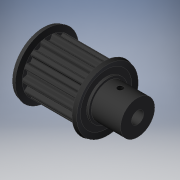
# Autodesk Inventor part: TTPA14T5200-B-P5_b
Saved by Autodesk Inventor 2019 (Build 230136000, 136)
## iProperties
Created: 2023-11-07
Part Number: TTPA14T5200-B-P5_b
Material: Generic
Catalog Web Link: www.cadenas.de
Description: TTPA__T5050, TTPA__T5100, TTPA__T5150, TTPA__T5200, TTPA__T5250, TTPB__T5050, TTPB__T5100, TTPB__T5150, TTPB__T5200, TTPB__T5250, TTPK__T5050, TTPK__T5100, TTPK__T5150, TTPK__T5200, TTPK__T5250, TTPN__T5050, TTPN__T5100, TTPN__T5150, TTPN__T5200, TTPN__T5250, TTPT__T5050, TTPT__T5100, TTPT__T5150, TTPT__T5200, TTPT__T5250, TTPM__T5050, TTPM__T5100, TTPM__T5150, TTPM__T5200, TTPM__T5250, TTPP__T5050, TTPP__T5100, TTPP__T5150, TTPP__T5200, TTPP__T5250, TTPS__T5050, TTPS__T5100, TTPS__T5150, TTPS__T5200, TTPS__T5250_b-Timing Pulleys T5 Type
Vendor: MISUMI
Document SubType Name: Modeling
Designer: psAdmin
Manufacturer: MISUMI
Mass: 9.71654 g
Surface Area: 50.0601 cm^2
Volume: 9.71654 cm^3
Density: 1 g/cm^3
Appearance: PSOLRGB-175-175-175
Category: PARTsolutions
Company: MISUMI
Title: TTPA14T5200-B-P5
Author: Cadenas PARTsolutions
Comments: Timing Pulleys T5 Type
PSOL_IDENT_0: {$CADENAS_DATA/23d-libs/misumi/metric/51_timing_pulleys/ttpt_t5/ttpa_t5.prj},938 {VTYP=3D},{NB=TTPA1
PSOL_IDENT_1: 4T5200-B-P5_b},{LINA=TTPA14T5200-B-P5},{NN=TTPA__T5050, TTPA__T5100, TTPA__T5150, TTPA__T5200, TTPA_
PSOL_IDENT_2: _T5250, TTPB__T5050, TTPB__T5100, TTPB__T5150, TTPB__T5200, TTPB__T5250, TTPK__T5050, TTPK__T5100, T
PSOL_IDENT_3: TPK__T5150, TTPK__T5200, TTPK__T5250, TTPN__T5050, TTPN__T5100, TTPN__T5150, TTPN__T5200, TTPN__T525
PSOL_IDENT_4: 0, TTPT__T5050, TTPT__T5100, TTPT__T5150, TTPT__T5200, TTPT__T5250, TTPM__T5050, TTPM__T5100, TTPM__
PSOL_IDENT_5: T5150, TTPM__T5200, TTPM__T5250, TTPP__T5050, TTPP__T5100, TTPP__T5150, TTPP__T5200, TTPP__T5250, TT
PSOL_IDENT_6: PS__T5050, TTPS__T5100, TTPS__T5150, TTPS__T5200, TTPS__T5250_b},{DATE=29.05.2023 09:16:51},{GEOMDAT
PSOL_IDENT_7: E=15.12.2022 08:47:30},{VERSION=},{LINEID=320},{WBVAR=MATP,ST,TNW,PS,SBS,DD,Z,J,Q,R,S,T,ALT1,ALT2,M,
PSOL_IDENT_8: QSC,QFC,QTC,ALT3,K,KSC,KFC,KTC,ALT4,ZM,ZSC,ZFC,ZTC,ALT5,ALT6,ALT7,FC,ALT8,SRG,ALT9,BTC,TL,ALT10,TPC,
PSOL_IDENT_9: ALT11,BC,ALT12,SLH,ALT13,BN},{WBNUMERIC=DD,Z,J,Q,R,S,T,QSC,QFC,QTC,K,KSC,KFC,KTC,ZSC,ZFC,ZTC,FC,SRG,
PSOL_IDENT_10: BTC,TL,BC,SLH,BN}  {NB=TTPA14T5200-B-P5_b},{LINA=TTPA14T5200-B-P5},{KT=DUMMY},{PN=TTPA14T5200-B-P5},
PSOL_IDENT_11: {TYPE=TTPA},{MATP=A2017},{MATPALG= 'A2017','Aluminum Alloy 2000 series','S45C','1045 Carbon Steel Eq
PSOL_IDENT_12: uivalent','SUS304','304 Stainless Steel' },{ST=CA},{STALG= 'CA','Clear Anodize','BA','Black Anodize'
PSOL_IDENT_13: ,'HAT','Hard Clear Anodize','ENP','Electroless Nickel Plating' },{NT=14},{TNW=T5200},{TNWALG= 'T5050'
PSOL_IDENT_14: , 'T5100' , 'T5150' , 'T5200' , 'T5250' },{BW=20},{PS=B},{PSALG= 'A','B' },{SBS=P},{SBSALG= 'H','Ro
PSOL_IDENT_15: und Hole','P','Round Hole + Tap','V','Stepped Hole','F','Stepped Hole (Counterbore holes on the boss
PSOL_IDENT_16: side)' },{DD=5.00},{DDALG=[5:6/1],6.35,[7:8/1]},{DDHA=},{DDPA=},{DDNA=},{DDCA=},{DDVA=},{DDY=},{DDW
PSOL_IDENT_17: B=},{DDHB=[5:6/1],6.35,[7:10/1]},{DDPB=[5:6/1],6.35,[7:8/1]},{DDNB=},{DDNK=[10:10/1]},{DDCB=},{DDVFB=
PSOL_IDENT_18: [5:6/1],6.35,[7:8/1]},{Z=0},{ZALG=[0]},{ZMIN=7.000},{ZAMAX=0.000},{ZBMAX=10.000},{DDZ=5.000},{J=0.0}
PSOL_IDENT_19: ,{JALG=[0]},{JMIN=2.000},{JMAX=37.000},{JPN=},{Q=0},{QALG=[0]},{QRMIN=7.000},{QRMAX=0.000},{WBQMIN=9
PSOL_IDENT_20: .000},{R=0},{RALG=[0]},{WBRMAX=-2.000},{S=0.0},{SALG=[0]},{SMAX=14.000},{T=0.0},{TALG=[0]},{TMAX=14.
PSOL_IDENT_21: 000},{SBSPN=-P5},{A=22},{W=27},{L=39},{PD=22.28},{OD=21.45},{D=14},{DALG=14.000},{DE=14.000},{F=26},
PSOL_IDENT_22: {E=16},{TT=1.6},{BBK=0.000},{TTK=0.000},{ALT1=},{ALT1ALG= '','w/o KC90 (Set Screw Angle)','KC90','wi
PSOL_IDENT_23: th KC90 (Set Screw Angle)' },{ANG=120.000},{ALT1PN=},{ALT2=},{ALT2ALG= '','Not applicable' },{M=N/A}
PSOL_IDENT_24: ,{MALG= 'N/A' },{MFTALG= 'N/A' },{MSALG= 'N/A' },{M3D=0.000},{KDML=0.000},{ML=0.000},{MUL=0.000},{PI
PSOL_IDENT_25: TCH=0.000},{QSC=0.0},{QSCALG=0},{QFC=0.0},{QFCALG=0},{QTC=0.0},{QTCALG=0},{QPCDMIN=0.000},{QPCDMINAL
PSOL_IDENT_26: G=0.000},{QPCDMAX=10.000},{ALT2PN=},{TAP=0.000},{ALT3=},{ALT3ALG= '','Not applicable' },{K=0.0},{KAL
PSOL_IDENT_27: G=0},{KMIN=4.000},{KFTMAX=0.000},{KSMAX=0.000},{KSC=0.0},{KSCALG=0},{KFC=0.0},{KFCALG=0},{KTC=0.0},{
PSOL_IDENT_28: KTCALG=0},{KSCMIN=9.000},{KPCDMIN=9.000},{KPCDMAX=10.000},{ALT3PN=},{ALT4=},{ALT4ALG= '','Not applic
PSOL_IDENT_29: able' },{ALT4MIN=15.500},{ALT4MAX=5.500},{ZM=N/A},{ZMALG= 'N/A' },{ZMFTALG= 'N/A' },{ZMSALG= 'N/A' }
PSOL_IDENT_30: ,{ZMDD1=0.0},{ZMDD2=0.0},{ZMHH=0.0},{ZSC=0.0},{ZSCALG=[0]},{ZFC=0.0},{ZFCALG=[0]},{ZTC=0.0},{ZTCALG=
PSOL_IDENT_31: [0]},{ZPCDMIN=0.000},{ZPCDMINALG=0.000},{ZPCDMAX=10.000},{ALT4PN=},{ALT5=},{ALT5ALG= '','w/o Flange
PSOL_IDENT_32: not Attached','NFC','with NFC (Flange not Attached)' },{ALT5PN=},{ALT6=},{ALT6ALG= '','w/o Flange At
PSOL_IDENT_33: tached on One Side Only','RFC','with RFC (Flange Attached on The Boss Side Only)','LFC','with LFC (F
PSOL_IDENT_34: lange Attached on The Opposite Side Only)' },{ALT6PN=},{ALT7=},{ALT7ALG= '','w/o FC (Flange Cut)','F
PSOL_IDENT_35: C','with FC (Flange Cut)' },{FC=0.0},{FCALG=0},{FCMIN=22.5},{FCMAX=24.0},{ALT7PN=},{ALT8=},{ALT8ALG=
PSOL_IDENT_36: '','Not applicable' },{ALT8ALGALG=10.000},{ALT8DD2=0.000},{ALT8MM=0.000},{ALT8NN=0.000},{QC=0.000},
PSOL_IDENT_37: {KC=0.000},{ZC=0.000},{SRG=0.0},{SRGALG=[0]},{SRGMAX=0.000},{SRGMAX1=0.000},{DD2=0.0},{MM=0.00},{NN=
PSOL_IDENT_38: 0.00},{ALT8PN=},{ALT9=},{ALT9ALG= '','Not applicable' },{BTC9=7.000},{TL9=1.000},{BTC=0},{BTCALG=[0]
PSOL_IDENT_39: },{TL=0.0},{TLALG=0},{TLMIN=1.000},{TLMAX=-27.500},{BTCL=0},{BTCD=0},{ALT9PN=},{WLBCTL=39.000},{ALT1
PSOL_IDENT_40: 0=},{ALT10ALG= '','w/o TPC (Tapped Hole Dimension)','TPC','with TPC (Tapped Hole Dimension)' },{TPC=
PSOL_IDENT_41: N/A},{TPCALG= 'N/A' },{TPCM=3.000},{ALT10PN=},{ALT11=},{ALT11ALG= '','w/o BC (Boss Cut)','BC','with
PSOL_IDENT_42: BC (Boss Cut)' },{BC=0.0},{BCALG=0},{BCMIN=6.000},{BCMAX=11.500},{M1WBC=32.000},{ALT11PN=},{KTT=4.50
PSOL_IDENT_43: 0},{ALT12=},{ALT12ALG= '','w/o SLH (Set Screw Length)','SLH','with SLH (Set Screw Length)' },{SLH=0}
PSOL_IDENT_44: ,{SLHALG=[0]},{ALT12PN=},{AC=M3x3},{M1=3.000},{M1L=3.000},{ALT811SRG3D=1.000},{ALT13=},{ALT13ALG= ''
PSOL_IDENT_45: ,'w/o BN (Hub Lengthening)','BN','with BN (Hub Lengthening)' },{BN=0.0},{BNALG=0},{BNMIN=12.5},{BNMA
PSOL_IDENT_46: X=22.0},{ALT13PN=}
NB: TTPA14T5200-B-P5_b
NN: 0
NT: 14
NBSYN: $PN._b
LINA: TTPA14T5200-B-P5
CATALOG: Misumi
PN: TTPA14T5200-B-P5
MATP: Aluminum Alloy 2000 series
ST: Clear Anodize
TNW: T5200
BW: 20
PS: B
SBS: Round Hole + Tap
DD: 5
Z: 0
J: 0
Q: 0
R: 0
S: 0
T: 0
A: 22
W: 27
L: 39
PD: 22.28
OD: 21.45
D: 14
F: 26
E: 16
TT: 1.6
ALT1: w/o KC90 (Set Screw Angle)
ALT2: Not applicable
M: N/A
QSC: 0
QFC: 0
QTC: 0
ALT3: Not applicable
K: 0
KSC: 0
KFC: 0
KTC: 0
ALT4: Not applicable
ZM: N/A
ZMDD1: 0
ZMDD2: 0
ZMHH: 0
ZSC: 0
ZFC: 0
ZTC: 0
ALT5: w/o Flange not Attached
ALT6: w/o Flange Attached on One Side Only
ALT7: w/o FC (Flange Cut)
FC: 0
ALT8: Not applicable
SRG: 0
DD2: 0
MM: 0
ALT9: Not applicable
BTC: 0
TL: 0
BTCL: 0
BTCD: 0
ALT10: w/o TPC (Tapped Hole Dimension)
TPC: N/A
ALT11: w/o BC (Boss Cut)
BC: 0
ALT12: w/o SLH (Set Screw Length)
SLH: 0
AC: M3x3
ALT13: w/o BN (Hub Lengthening)
BN: 0
SUPPLIER: MISUMI
ARTICLENO: TTPA14T5200-B-P5_b
BOMINFO: TTPA14T5200-B-P5
CREATOR: CADENAS GmbH
Autodesk Inventor part; units mm, degrees
note: some values were not read from the file. Chosen so that the rebuilt part matches the saved one: pattern direction of "Circular Pattern1".
sketch "_____3" plane through (0, 0, 0) normal (0, 0, 1) x (1, 0, 0)
  line L0 (39, 0) -> (0, 0)
  line L1 (0, 0) -> (0, 8)
  line L2 (0, 8) -> (0.9, 8)
  line L3 (0.9, 8) -> (0.9, 10.5144)
  line L4 (0.9, 10.5144) -> (0.3449, 12.5859)
  line L5 (0.3449, 12.5859) -> (1.8904, 13)
  line L6 (1.8904, 13) -> (2.5, 10.725)
  line L7 (2.5, 10.725) -> (24.5, 10.725)
  line L8 (24.5, 10.725) -> (25.1096, 13)
  line L9 (25.1096, 13) -> (26.6551, 12.5859)
  line L10 (26.6551, 12.5859) -> (26.1, 10.5144)
  line L11 (26.1, 10.5144) -> (26.1, 8)
  line L12 (26.1, 8) -> (27, 8)
  line L13 (27, 8) -> (27, 7)
  line L14 (27, 7) -> (39, 7)
  line L15 (39, 7) -> (39, 0)
  line L16 (39, 0) -> (0, 0)
  constraints: 34 end point
revolve "Revolution1" add sketch "_____3" angle 360 about axis through (39, 0, 0) along (1, 0, 0)
sketch "Sketch2" plane through (39, 0, 0) normal (1, 0, 0) x (0, 0, -1)
  point P0 (0, 0)
hole "Hole1" at (39, 0, 0) direction (-1, 0, 0) diameter 5 depth 39
sketch "_____6" plane through (2.5, 0, 0) normal (1, 0, 0) x (0, 0, -1)
  line L0 (-2.0929, 10.9416) -> (-2.015, 10.534)
  arc A0 (-1.3585, 10.1983) -> (-2.015, 10.534) centre (-1.9022, 9.9447) ccw
  line L1 (-1.3585, 10.1983) -> (-0.8661, 9.1423)
  arc A1 (-0.8661, 9.1423) -> (-0.4819, 8.912) centre (-0.5035, 9.3114) ccw
  arc A2 (0.4819, 8.912) -> (-0.4819, 8.912) centre (0, 0) ccw
  arc A3 (0.4819, 8.912) -> (0.8661, 9.1423) centre (0.5035, 9.3114) ccw
  line L2 (0.8661, 9.1423) -> (1.3585, 10.1983)
  arc A4 (2.015, 10.534) -> (1.3585, 10.1983) centre (1.9022, 9.9447) ccw
  line L3 (2.015, 10.534) -> (2.0929, 10.9416)
  arc A5 (2.0929, 10.9416) -> (-2.0929, 10.9416) centre (0, 0) ccw
  constraints: 12 point on circle, 8 end point, 6 centre point
extrude "Extrusion1" cut sketch "_____6" along normal blind 22
pattern_circular "Circular Pattern1" count 14 over 360 about axis through (2.5, 0, 0) along (1, 0, 0) of "Extrusion1"
sketch "_____17" plane through (32, 0, 0) normal (1, 0, 0) x (0, 0, -1)
  line L0 (0, 0) -> (0, 7)
  line L1 (0, 7) -> (1.2295, 7)
  line L2 (1.2295, 7) -> (1.2295, 0)
  line L3 (1.2295, 0) -> (0, 0)
  line L4 (0, 0) -> (0, 7)
  constraints: 10 end point
revolve "Revolution2" cut sketch "_____17" angle 360 about axis through (32, 0, 0) along (0, -1, 0)
thread "Thread1" size "M3x0.5" class "6H" standard "ISO Metric profile" length 4.5
sketch "_____18" plane through (32, 0, 0) normal (1, 0, 0) x (0, 0, -1)
  line L0 (0, 0) -> (6.0622, -3.5)
  line L1 (6.0622, -3.5) -> (5.4474, -4.5648)
  line L2 (5.4474, -4.5648) -> (-0.6148, -1.0648)
  line L3 (-0.6148, -1.0648) -> (0, 0)
  line L4 (0, 0) -> (6.0622, -3.5)
  constraints: 10 end point
revolve "Revolution3" cut sketch "_____18" angle 360 about axis through (32, 0, 0) along (0, 0.5, 0.8660254)
thread "Thread2" size "M3x0.5" class "6H" standard "ISO Metric profile" length 4.5 offset 0.2144
ref_plane "to_screw1_XY" through (32, 2.5, 0) normal (0, 1, 0) x (1, 0, 0)
ref_plane "to_screw1_YZ" through (32, 2.5, 0) normal (1, 0, 0) x (0, 0, -1)
ref_plane "to_screw1_ZX" through (32, 2.5, 0) normal (0, 0, -1) x (0, 1, 0)
ref_plane "to_screw2_XY" through (32, -1.25, -2.1651) normal (0, -0.5, -0.8660254) x (1, 0, 0)
ref_plane "to_screw2_YZ" through (32, -1.25, -2.1651) normal (1, 0, 0) x (0, -0.8660254, 0.5)
ref_plane "to_screw2_ZX" through (32, -1.25, -2.1651) normal (0, -0.8660254, 0.5) x (0, -0.5, -0.8660254)
body "Solid1"
